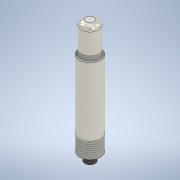
# Autodesk Inventor part: W504
Saved by Autodesk Inventor 2020 (Build 240168000, 168)
## iProperties
Created: 2021-10-16
Part Number: W504
Material: Genérico
Document SubType Name: Modeling
Designer: DANIEL
Density: 1 g/cm^3
Appearance: Valor por defecto
Author: DANIEL
Autodesk Inventor part; units mm, degrees
ref_plane "YZ Plane" through (0, 0, 0) normal (1, 0, 0) x (0, 1, 0)
ref_plane "XZ Plane" through (0, 0, 0) normal (0, 1, 0) x (-1, 0, 0)
ref_plane "XY Plane" through (0, 0, 0) normal (0, 0, 1) x (1, 0, 0)
sketch "Boceto1" plane through (0, 0, 0) normal (0, 1, 0) x (-1, 0, 0)
  circle A0 centre (0, 0) radius 13
  dimension "d0" = 26
  constraints: 1 centre point, 1 coincident
  measures "d0" diameter of A0
extrude "Extrusión1" add sketch "Boceto1" along normal blind 151
sketch "Boceto2" plane through (0, 151, 0) normal (0, 1, 0) x (1, 0, 0)
  circle A0 centre (0, 0) radius 10.75
  circle A1 centre (0, 0) radius 13
  dimension "d3" = 21.5
  constraints: 2 centre point, 2 coincident
  measures "d3" diameter of A0
extrude "Extrusión2" cut sketch "Boceto2" against normal blind 37.2
fillet "Empalme1" radius 6 1 edges at (-10.75, 151, 0)
thread "Rosca1" size "3/4" designation "3/4 - 14 NPT" standard "NPT" length 31.2 offset 25
sketch "Boceto3" plane through (0, 0, 0) normal (0, -1, 0) x (1, 0, 0)
  circle A0 centre (0, 0) radius 6.5
  circle A1 centre (0, 0) radius 13
  dimension "d9" = 13
  constraints: 2 centre point, 2 coincident
  measures "d9" diameter of A0
extrude "Extrusión3" cut sketch "Boceto3" against normal blind 10
sketch "Boceto4" plane through (0, 10, 0) normal (0, -1, 0) x (1, 0, 0)
  circle A0 centre (0, 0) radius 13
  circle A1 centre (0, 0) radius 12.95
  dimension "d12" = 25.9
  constraints: 2 centre point, 2 coincident
  measures "d12" diameter of A1
extrude "Extrusión4" cut sketch "Boceto4" against normal blind 20
thread "Rosca2" size "1/4" designation "1/4 - 18 NPT" standard "NPT" length 15.103
thread "Rosca3" size "1" designation "1 - 11.5 NPT" standard "NPT" length 25.006 offset 1
